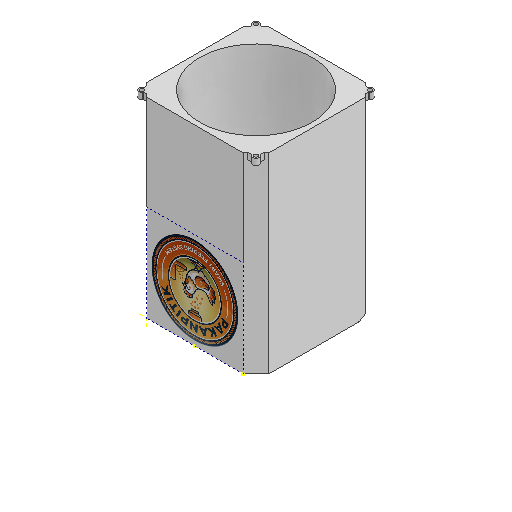
# Autodesk Inventor part: Tank
Saved by Autodesk Inventor 2026.2 (Build 302298010, 298A)
## iProperties
Created: 2026-05-23
Part Number: Tank
Material: Generic
Document SubType Name: Modeling
Designer: rizky
Density: 1 g/cm^3
Appearance: Default
Author: rizky
Autodesk Inventor part; units mm, degrees
ref_plane "YZ Plane" through (0, 0, 0) normal (1, 0, 0) x (0, 1, 0)
ref_plane "XZ Plane" through (0, 0, 0) normal (0, 1, 0) x (-1, 0, 0)
ref_plane "XY Plane" through (0, 0, 0) normal (0, 0, 1) x (1, 0, 0)
sketch "Sketch1" plane through (0, 0, 0) normal (0, 1, 0) x (-1, 0, 0)
  circle A0 centre (0, 0) radius 43.732
  line L0 (-47.5, -47.5) -> (47.5, -47.5)
  line L1 (47.5, -47.5) -> (47.5, 47.5)
  line L2 (47.5, 47.5) -> (-47.5, 47.5)
  line L3 (-47.5, 47.5) -> (-47.5, -47.5)
  line L4 (-47.5, -47.5) -> (47.5, 47.5) construction
  line L5 (47.5, -47.5) -> (-47.5, 47.5) construction
  dimension "d0" = 87.464
  dimension "d4" = 95
  dimension "d5" = 95
  constraints: 12 end point, 2 midpoint, 2 parallel, 1 centre point, 1 coincident, 1 horizontal, 1 perpendicular
  measures "d0" diameter of A0
  measures "d4" distance of L2.end L1.end
  measures "d5" distance of L1.end L0.end
extrude "Extrusion1" add sketch "Sketch1" along normal blind 149
chamfer "Chamfer1" distance 10 angle 45 4 edges at (47.5, 74.5, -47.5) (47.5, 74.5, 47.5) (-47.5, 74.5, 47.5) (-47.5, 74.5, -47.5)
sketch "Sketch2" plane through (0, 149, 0) normal (0, 1, 0) x (1, 0, 0)
  line L0 (-47.5, 37.5) -> (-37.5, 47.5) projected
  line L1 (-47.5, 37.5) -> (-47.5, -37.5) projected
  line L2 (-37.5, -47.5) -> (-47.5, -37.5) projected
  line L3 (-37.5, -47.5) -> (37.5, -47.5) projected
  line L4 (47.5, -37.5) -> (37.5, -47.5) projected
  line L5 (47.5, -37.5) -> (47.5, 37.5) projected
  line L6 (37.5, 47.5) -> (47.5, 37.5) projected
  line L7 (37.5, 47.5) -> (-37.5, 47.5) projected
  circle A0 centre (0, 0) radius 43.732 projected
  line L8 (-42.5, 42.5) -> (-44.3434, 44.3434)
  circle A1 centre (-44.3434, 44.3434) radius 1.5
  circle A2 centre (-44.3434, 44.3434) radius 2.5
  line L9 (-42.5757, 46.1112) -> (-40.7322, 44.2678)
  line L10 (-46.1112, 42.5757) -> (-44.2678, 40.7322)
  line L11 (0, 47.5) -> (0, 44.5)
  line L12 (-47.5, 0) -> (-44.5, 0)
  circle A3 centre (44.3434, 44.3434) radius 1.5
  circle A4 centre (44.3434, 44.3434) radius 2.5
  line L13 (42.5757, 46.1112) -> (40.7322, 44.2678)
  line L14 (46.1112, 42.5757) -> (44.2678, 40.7322)
  circle A5 centre (-44.3434, -44.3434) radius 1.5
  circle A6 centre (-44.3434, -44.3434) radius 2.5
  line L15 (-42.5757, -46.1112) -> (-40.7322, -44.2678)
  line L16 (-46.1112, -42.5757) -> (-44.2678, -40.7322)
  circle A7 centre (44.3434, -44.3434) radius 2.5
  circle A8 centre (44.3434, -44.3434) radius 1.5
  line L17 (42.5757, -46.1112) -> (40.7322, -44.2678)
  line L18 (46.1112, -42.5757) -> (44.2678, -40.7322)
  dimension "d9" = 2.607
  dimension "d10" = 3
  dimension "d11" = 1
  dimension "d12" = 3
  dimension "d13" = 3
  constraints: 22 end point, 17 symmetric about line, 4 centre point, 3 horizontal, 3 midpoint, 2 vertical, 1 coincident, 1 perpendicular, 1 point on line, 16 other
  measures "d9" distance of L8.start L8.end
  measures "d10" diameter of A1
  measures "d12" distance of L11.start L11.end
  measures "d13" distance of L12.start L12.end
extrude "Extrusion2" add sketch "Sketch2" against normal blind 5 contours L10 A2 L8 L0 | L8 A2 L9 L0 | A2 | L2 L15 A6 L16 | A6 | L13 A4 L14 L6 | L4 L18 A7 L17 | A4 | A7
fillet "Fillet1" radius 2 8 edges at (44.2678, 146.5, -40.7322) (40.7322, 146.5, -44.2678) (44.2678, 146.5, 40.7322) (40.7322, 146.5, 44.2678) (-40.7322, 146.5, 44.2678) (-44.2678, 146.5, 40.7322) (-44.2678, 146.5, -40.7322) (-40.7322, 146.5, -44.2678)
sketch "Sketch5" plane through (0, 0, 0) normal (0, -1, 0) x (1, 0, 0)
  line L0 (-37.5, -47.5) -> (-47.5, -37.5) projected
  line L1 (37.5, -47.5) -> (-37.5, -47.5) projected
  line L2 (47.5, -37.5) -> (37.5, -47.5) projected
  line L3 (47.5, 37.5) -> (47.5, -37.5) projected
  line L4 (37.5, 47.5) -> (47.5, 37.5) projected
  line L5 (-37.5, 47.5) -> (37.5, 47.5) projected
  line L6 (-47.5, 37.5) -> (-37.5, 47.5) projected
  line L7 (-47.5, -37.5) -> (-47.5, 37.5) projected
  circle A0 centre (0, 0) radius 43.732 projected
  circle A1 centre (0, 0) radius 43.732 projected
  line L8 (0, -43.732) -> (0, -38.732)
  line L9 (-20.3057, -38.732) -> (20.3057, -38.732)
  dimension "d30" = 5
  constraints: 4 end point, 3 point on circle, 1 horizontal, 1 midpoint, 1 vertical
  measures "d30" distance of L8.start L8.end
extrude "Extrusion4" add sketch "Sketch5" against normal blind 25 contours L9 L8 A0 | A0 L8 L9
sketch "Sketch6" plane through (37.5, 0, -47.5) normal (0, 0, -1) x (-1, 0, 0)
  line L0 (0, 0) -> (75, 0) projected
  line L1 (37.5, 0) -> (37.5, 15)
  line L2 (37.5, 15) -> (25, 15)
  circle A0 centre (25, 15) radius 2.5
  circle A1 centre (50, 15) radius 2.5
  dimension "d31" = 15
  dimension "d32" = 12.5
  dimension "d33" = 5
  constraints: 4 end point, 2 centre point, 1 coincident, 1 horizontal, 1 symmetric about line, 1 vertical, 1 other
  measures "d31" distance of L1.start L1.end
  measures "d32" distance of L1.end L2.end
  measures "d33" diameter of A0
extrude "Extrusion5" cut sketch "Sketch6" against normal blind 30
sketch "Sketch7" plane through (-47.5, 0, -37.5) normal (-1, 0, 0) x (0, 0, 1)
  line L0 (0, 0) -> (0, 149) projected
  line L1 (0, 0) -> (75, 0) projected
  line L2 (75, 149) -> (75, 0) projected
  line L3 (0, 149) -> (75, 149) projected
  line L4 (-8.182, 149) -> (-8.182, 144) projected
  line L5 (-8.182, 149) -> (-10, 149) projected
  line L6 (-10, 149) -> (-10, 0) projected
  line L7 (-10, 0) -> (0, 0) projected
  line L8 (0, 0) -> (0, 149) projected
  line L9 (0, 149) -> (-1.818, 149) projected
  line L10 (-1.818, 144) -> (-1.818, 149) projected
  line L11 (-1.818, 144) -> (-8.182, 144) projected
  line L12 (0, 149) -> (0, 0) projected
  line L13 (0, 0) -> (14.1421, 0) construction
  line L14 (-10, 0) -> (5, 0)
  line L15 (5, 0) -> (-10, 8.6603)
  point P0 (37.5, 0)
  dimension "d39" = 15
  dimension "d40" = 30
  constraints: 6 end point, 2 point on line, 1 horizontal
  measures "d39" distance of L6.end L14.end
  measures "d40" angle of L14 L15
extrude "Extrusion7" cut sketch "Sketch7" against normal through all contours L7 L6 L15 L0 | L0 L15 L1
sketch "Sketch8" plane through (-37.5, 0, 47.5) normal (0, 0, 1) x (1, 0, 0)
  line L0 (75, 0) -> (0, 0) construction
  line L1 (0, 0) -> (0, 75) construction
  line L2 (0, 75) -> (75, 75) construction
  line L3 (75, 75) -> (75, 0) construction
  point P0 (37.5, 0)
  dimension "d0" = 87.464
  dimension "d4" = 95
  dimension "d5" = 95
  constraints: 2 coincident, 2 other
body "Solid1"
